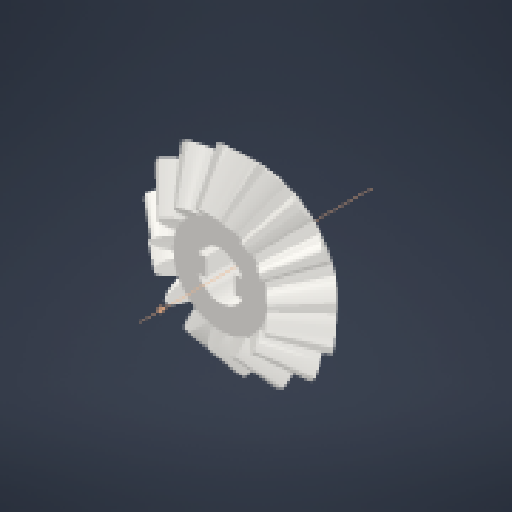
# Autodesk Inventor part: Bevel Gear2
Saved by Autodesk Inventor 2026 (Build 300175050, 175E)
## iProperties
CustomPartVersion: 1
Created: 2026-04-30
Part Number: Bevel Gear2
Material: Steel, Mild
Document SubType Name: Modeling
Designer: sniel
Categories: <?xml version="1.0" encoding="UTF-16"?> <MemberInstance><Categories><FamilyTemplate><FamilyTemplateParameter ValueType="xs:double" Id="1" ObjectReferenceKey="da_z" ObjectType="kUserParameterObject"/><FamilyTemplateParameter ValueType="xs:double" Id="2" ObjectReferenceKey="da_b" ObjectType="kUserParameterObject"/><FamilyTemplateParameter ValueType="xs:double" Id="3" ObjectReferenceKey="da_beta" ObjectType="kUserParameterObject"/><FamilyTemplateParameter ValueType="xs:double" Id="4" ObjectReferenceKey="da_dae" ObjectType="kUserParameterObject"/><FamilyTemplateParameter ValueType="xs:double" Id="5" ObjectReferenceKey="da_ve" ObjectType="kUserParameterObject"/><FamilyTemplateParameter ValueType="xs:double" Id="6" ObjectReferenceKey="da_omega" ObjectType="kUserParameterObject"/><FamilyTemplateParameter ValueType="xs:string" Id="7" ObjectReferenceKey="EAIAABAAAAAAHwAAAAAAAIAAAAAAAAAA" ObjectType="83914240" SubObjectId="SurfaceGeometry"/></FamilyTemplate><ParamToTemplateMap><ParamToTemplate CategoryParameter="//CategoryParameter[@InternalName='046C89C9-8512-4d59-83FE-43B91F4F132A']" TemplateParameter="1"/><ParamToTemplate CategoryParameter="//CategoryParameter[@InternalName='2552DF32-E462-4b46-AEBF-C6C7768E72AC']" TemplateParameter="2"/><ParamToTemplate CategoryParameter="//CategoryParameter[@InternalName='C9EE641D-15FC-4fae-A226-E94C4372FDD7']" TemplateParameter="3"/><ParamToTemplate><ParamToTemplate CategoryParameter="//CategoryParameter[@InternalName='00B6519A-459B-49c7-AD84-2E56D39A5744']" ConstantValue="-0.000000"/></ParamToTemplate><ParamToTemplate><ParamToTemplate CategoryParameter="//CategoryParameter[@InternalName='04B31F0E-C7A6-4894-AA32-9629BEFACF47']" ConstantValue="1.000000"/></ParamToTemplate><ParamToTemplate><ParamToTemplate CategoryParameter="//CategoryParameter[@InternalName='43CBEC2E-7847-49e7-A936-2F7889FCB2D9']" ConstantValue="0.200000"/></ParamToTemplate><ParamToTemplate><ParamToTemplate CategoryParameter="//CategoryParameter[@InternalName='B1EFC894-105D-4ebd-86BF-FA20ED196853']" ConstantValue="0.300000"/></ParamToTemplate><ParamToTemplate><ParamToTemplate CategoryParameter="//CategoryParameter[@InternalName='51175063-3D10-4879-93E8-6246FE8B403D']" ConstantValue="2060000000.000000"/></ParamToTemplate><ParamToTemplate><ParamToTemplate CategoryParameter="//CategoryParameter[@InternalName='A3A52E27-4454-46a9-B0BD-C932399B70AF']" ConstantValue="0.300000"/></ParamToTemplate><ParamToTemplate CategoryParameter="//CategoryParameter[@InternalName='2A200944-5A8C-41ca-B96E-8520D2E510F1']" TemplateParameter="4"/><ParamToTemplate><ParamToTemplate CategoryParameter="//CategoryParameter[@InternalName='1A637F62-92C8-44bc-B81F-10802510B579']" ConstantValue="1.982903"/></ParamToTemplate><ParamToTemplate CategoryParameter="//CategoryParameter[@InternalName='B52DD4BE-6863-48fb-BF58-89EF6F9EC65C']" TemplateParameter="5"/><ParamToTemplate><ParamToTemplate CategoryParameter="//CategoryParameter[@InternalName='3956BFF2-84D2-457d-93C2-9B0613DEBA67']" ConstantValue="0.820609"/></ParamToTemplate><ParamToTemplate CategoryParameter="//CategoryParameter[@InternalName='739CFA02-461B-4bf8-8049-181FCAD8B28F']" TemplateParameter="6"/><ParamToTemplate><ParamToTemplate CategoryParameter="//CategoryParameter[@InternalName='A27E999F-E2CE-4481-8A2A-EBF499C4C3C5']" ConstantValue="-0.000000"/></ParamToTemplate><ParamToTemplate><ParamToTemplate CategoryParameter="//CategoryParameter[@InternalName='9E1B4470-B2D3-4ff1-B813-535BB4CDF51A']" ConstantValue="3520000.000000"/></ParamToTemplate><ParamToTemplate><ParamToTemplate CategoryParameter="//CategoryParameter[@InternalName='F8452263-BFF6-458c-9FB1-07C4B99E95CD']" ConstantValue="11400000.000000"/></ParamToTemplate><ParamToTemplate><ParamToTemplate CategoryParameter="//CategoryParameter[@InternalName='3E3BB259-FD49-497f-8171-6EBC954A3479']" ConstantValue="2.000000"/></ParamToTemplate><ParamToTemplate CategoryParameter="//CategoryParameter[@InternalName='27C3BAF2-7550-4e4b-AE2C-0DB134B7D9B7']" TemplateParameter="7"/></ParamToTemplateMap><Category DisplayName="Gear" InternalName="DC85795E-93AB-48d5-8EEE-5A27447B64BD" Mnemonic="Gear"><CategoryParameter DisplayName="z" InternalName="046C89C9-8512-4d59-83FE-43B91F4F132A" Mnemonic="z"/><CategoryParameter DisplayName="b" InternalName="2552DF32-E462-4b46-AEBF-C6C7768E72AC" Mnemonic="b"/><CategoryParameter DisplayName="||b|" InternalName="C9EE641D-15FC-4fae-A226-E94C4372FDD7" Mnemonic="beta"/><CategoryParameter DisplayName="x" InternalName="00B6519A-459B-49c7-AD84-2E56D39A5744" Mnemonic="x"/><CategoryParameter DisplayName="a*" InternalName="04B31F0E-C7A6-4894-AA32-9629BEFACF47" Mnemonic="a"/><CategoryParameter DisplayName="c*" InternalName="43CBEC2E-7847-49e7-A936-2F7889FCB2D9" Mnemonic="c"/><CategoryParameter DisplayName="r|.f|*" InternalName="B1EFC894-105D-4ebd-86BF-FA20ED196853" Mnemonic="rf"/><CategoryParameter DisplayName="E" InternalName="51175063-3D10-4879-93E8-6246FE8B403D" Mnemonic="E"/><CategoryParameter DisplayName="||m|" InternalName="A3A52E27-4454-46a9-B0BD-C932399B70AF" Mnemonic="mi"/><Category DisplayName="BevelGear" InternalName="0C98F69A-0C2B-4791-B2FE-7691BB227E77" Mnemonic="BevelGear"><CategoryParameter DisplayName="d|.ae|" InternalName="2A200944-5A8C-41ca-B96E-8520D2E510F1" Mnemonic="dae"/><CategoryParameter DisplayName="d|.ai|" InternalName="1A637F62-92C8-44bc-B81F-10802510B579" Mnemonic="dai"/><CategoryParameter DisplayName="A|.e|" InternalName="B52DD4BE-6863-48fb-BF58-89EF6F9EC65C" Mnemonic="ve"/><CategoryParameter DisplayName="A|.i|" InternalName="3956BFF2-84D2-457d-93C2-9B0613DEBA67" Mnemonic="vi"/><CategoryParameter DisplayName="||S|" InternalName="739CFA02-461B-4bf8-8049-181FCAD8B28F" Mnemonic="omega"/><CategoryParameter DisplayName="x|.t|" InternalName="A27E999F-E2CE-4481-8A2A-EBF499C4C3C5" Mnemonic="xt"/><CategoryParameter DisplayName="||s||.Flim|" InternalName="9E1B4470-B2D3-4ff1-B813-535BB4CDF51A" Mnemonic="sFlim"/><CategoryParameter DisplayName="||s||.Hlim|" InternalName="F8452263-BFF6-458c-9FB1-07C4B99E95CD" Mnemonic="sHlim"/><CategoryParameter DisplayName="type" InternalName="3E3BB259-FD49-497f-8171-6EBC954A3479" Mnemonic="type"/><CategoryParameter DisplayName="PitchDiameter" InternalName="27C3BAF2-7550-4e4b-AE2C-0DB134B7D9B7" Mnemonic="IDS_PITCHDIAM"/></Category></Category></Categories></MemberInstance>
Mass: 60.9118 g
Surface Area: 34.3074 cm^2
Volume: 7.7496 cm^3
Density: 7.86 g/cm^3
Appearance: Steel
Author: sniel
Autodesk Inventor part; units mm, degrees
ref_plane "Mesh Plane2" through (0, 0, 0) normal (0.9781476, 0.2079117, 0) x (0, 0, 1)
sketch "Teeth Body Sketch" plane through (0, 0, 0) normal (1, 0, 0) x (0, 1, 0)
  line L0 (0, 0) -> (13.302944, -16.697056) construction
  line L1 (13.302944, -16.697056) -> (16.414214, -13.585786)
  line L2 (16.414214, -13.585786) -> (0, 0) construction
  line L3 (15, -15) -> (0, 0) construction
  line L4 (8.035247, -10.085359) -> (9.914517, -8.206089)
  line L5 (13.302944, -16.697056) -> (8.035247, -10.085359)
  line L6 (16.414214, -13.585786) -> (9.914517, -8.206089)
  line L7 (0, -39.386751) -> (0, 6.564458)
  line L8 (0, -15) -> (16.414214, -15) construction
  dimension "d0" = 30
  dimension "d1" = 26.60589
  dimension "d2" = 32.82843
  dimension "d3" = 8.4
  dimension "d4" = 13.58579
  constraints: 16 end point, 4 point on line, 3 perpendicular, 2 collinear, 1 horizontal alignment, 1 vertical alignment
  measures "d0" diameter of L3.start L7
  measures "d1" diameter of L0.end L7
  measures "d2" diameter of L1.end L7
  measures "d3" distance between parallel lines of L1 L4
  measures "d4" vertical distance of L1.end L0.start
revolve "Teeth Body" add sketch "Teeth Body Sketch" angle 360 about axis through (0, 0, 0) along (0, 0, 1)
ref_plane "Tooth Plane" through (0, 15, -15) normal (0, -0.7071068, 0.7071068) x (1, 0, 0)
sketch "Start Sketch" plane through (0, 15, -15) normal (0, -0.7071068, 0.7071068) x (1, 0, 0)
  line L0 (0, -23.505131) -> (0, 10.644758)
  arc A0 (-0.859413, -2.928) -> (-4.075674, 2.979088) centre (-8.774532, -3.408453) ccw
  arc A1 (4.075674, 2.979088) -> (0.859413, -2.928) centre (8.774532, -3.408453) ccw
  line L1 (-0.859413, -2.928) -> (0.859413, -2.928)
  arc A2 (4.075674, 2.979088) -> (-4.075674, 2.979088) centre (0, -21.213203) ccw
  dimension "d7" = 7.92969
  dimension "d8" = 8.77453
  dimension "d9" = 17.80475
  dimension "d57" = 24.5332
  dimension "d58" = 18.2852
  constraints: 6 point on circle, 3 centre point, 3 symmetric about line, 2 end point, 1 coincident, 1 perpendicular, 1 other
  measures "d7" radius of A0
  measures "d8" horizontal distance of point (0, -21.213) A0.centre
  measures "d9" vertical distance of point (0, -21.213) A0.centre
  measures "d57" radius of A2
  measures "d58" distance from line of A2.centre L1
sketch "End Sketch" plane through (0, 8.90474, -8.90474) normal (0, -0.7071068, 0.7071068) x (1, 0, 0)
  line L0 (0, -15.35404) -> (0, 6.953444)
  arc A0 (-0.51019, -1.738205) -> (-2.419521, 1.768533) centre (-5.208995, -2.023426) ccw
  arc A1 (2.419521, 1.768533) -> (0.51019, -1.738205) centre (5.208995, -2.023426) ccw
  line L1 (-0.51019, -1.738205) -> (0.51019, -1.738205)
  arc A2 (2.419521, 1.768533) -> (-2.419521, 1.768533) centre (0, -12.593203) ccw
  dimension "d12" = 4.70745
  dimension "d15" = 5.20899
  dimension "d16" = 10.56978
  dimension "d59" = 14.56412
  dimension "d60" = 10.855
  constraints: 6 point on circle, 3 centre point, 3 symmetric about line, 2 end point, 1 coincident, 1 other
  measures "d12" radius of A0
  measures "d15" horizontal distance of A0.centre point (0, -12.593)
  measures "d16" vertical distance of A0.centre point (0, -12.593)
  measures "d59" radius of A2
  measures "d60" distance from line of A2.centre L1
loft "Loft" cut profiles "Start Sketch", "End Sketch"
pattern_circular "Circular Pattern" count 15 over 360 about axis through (0, 0, 0) along (0, 0, 1) of "Loft"
ref_plane "End Plane" through (0, 8.90474, -8.90474) normal (0, -0.7071068, 0.7071068) x (1, 0, 0)
sketch3d "3D Sketch Right"
ref_plane "End Plane Right" through (-2.29609, 8.603625, -8.90474) normal (0.1823277, -0.6831959, 0.7071068) x (0.9661849, 0.2578504, 0)
sketch "End Sketch Right" plane through (-2.29609, 8.603625, -8.90474) normal (0.1823277, -0.6831959, 0.7071068) x (0.9661849, 0.2578504, 0)
  arc A0 (-0.51019, -1.738205) -> (-2.419521, 1.768533) centre (-5.208995, -2.023426) ccw
  line L0 (0, -19.114994) -> (0, 10.288445)
  arc A1 (2.419521, 1.768533) -> (0.51019, -1.738205) centre (5.208995, -2.023426) ccw
  line L1 (-0.51019, -1.738205) -> (0.51019, -1.738205)
  arc A2 (2.419521, 1.768533) -> (-2.419521, 1.768533) centre (0, -12.593203) ccw
  dimension "d70" = 5.20899
  dimension "d71" = 10.56978
  dimension "d72" = 4.70745
  dimension "d73" = 10.855
  dimension "d74" = 14.56412
  constraints: 6 point on circle, 3 centre point, 3 symmetric about line, 2 end point, 1 coincident, 1 perpendicular, 1 other
  measures "d70" horizontal distance of A2.centre A0.centre
  measures "d71" vertical distance of point (0, -12.593) A0.centre
  measures "d72" radius of A0
  measures "d73" distance from line of point (0, -12.593) L1
  measures "d74" radius of A2
feature "Loft Right" [suppressed]
pattern_circular "Circular Pattern Right" [suppressed]
sketch3d "3D Sketch Left"
ref_plane "End Plane Left" through (2.297938, 8.603625, -8.905436) normal (-0.1824624, -0.6831509, 0.7071155) x (0.9661332, -0.258044, 0)
sketch "End Sketch Left" plane through (2.297938, 8.603625, -8.905436) normal (-0.1824624, -0.6831509, 0.7071155) x (0.9661332, -0.258044, 0)
  line L0 (0, -32.194268) -> (0, 15.171544)
  arc A0 (-0.51019, -1.73805) -> (-2.419521, 1.768689) centre (-5.208995, -2.02327) ccw
  arc A1 (2.419521, 1.768689) -> (0.51019, -1.73805) centre (5.208995, -2.02327) ccw
  line L1 (-0.51019, -1.73805) -> (0.51019, -1.73805)
  ellipse E0 centre (0, -5.80251) end of major axis (9.914517, -5.80251) minor radius 7.010708
  arc A2 (2.419521, 1.768689) -> (-2.419521, 1.768689) centre (0, -12.593048) ccw
  dimension "d56" = 7.01071
  dimension "d30" = 4.70745
  dimension "d31" = 5.20899
  dimension "d32" = 10.56978
  dimension "d61" = 14.56412
  dimension "d62" = 10.855
  constraints: 6 point on circle, 3 centre point, 3 symmetric about line, 2 end point, 1 coincident, 2 other
  measures "d30" radius of A0
  measures "d31" horizontal distance of point (0, -12.593) A0.centre
  measures "d32" vertical distance of A0.centre point (0, -12.593)
  measures "d61" radius of A2
  measures "d62" distance from line of point (0, -12.593) L1
feature "Loft Left" [suppressed]
pattern_circular "Circular Pattern Left" [suppressed]
sketch "Body Sketch" plane through (0, 0, 0) normal (1, 0, 0) x (0, 1, 0)
  line L0 (0, -35.037536) -> (0, -19.530831)
  line L1 (13.302944, -16.697056) -> (8.035247, -10.085359)
  line L2 (8.035247, -10.085359) -> (0, -10.085359)
  line L3 (13.302944, -16.697056) -> (0, -16.697056)
  constraints: 4 end point, 2 perpendicular, 2 point on line
sketch "Body Sketch outline for Fix Body" plane through (0, 0, 0) normal (1, 0, 0) x (0, 1, 0)
  line L0 (0, -16.697056) -> (13.302944, -16.697056)
  line L1 (0, -10.085359) -> (0, -16.697056)
  line L2 (8.035247, -10.085359) -> (0, -10.085359)
  line L3 (13.302944, -16.697056) -> (8.035247, -10.085359)
revolve "Fix Body" add sketch "Body Sketch outline for Fix Body" angle 360 about axis through (0, 0, 0) along (0, 0, 1)
sketch "Sketch6" plane through (0, 0, 0) normal (1, 0, 0) x (0, 1, 0)
  line L0 (15, -15) -> (0, 0)
  line L1 (0, -37.799919) -> (0, 6.299986)
surface revolve "Pitch Diameter" sketch "Sketch6" angle 360 about axis through (0, 0, 0) along (0, 0, 1) shown no curves L0
sketch "Sketch8" plane through (0, 0, -16.697056) normal (0, 0, -1) x (-1, 0, 0)
  circle A0 centre (0, 0) radius 4
  line L0 (-5.5, -1.5) -> (-2.5, -1.5)
  line L1 (-2.5, -1.5) -> (-2.5, 1.5)
  line L2 (-2.5, 1.5) -> (-5.5, 1.5)
  line L3 (-5.5, 1.5) -> (-5.5, -1.5)
  line L4 (-5.5, -1.5) -> (-2.5, 1.5) construction
  line L5 (-2.5, -1.5) -> (-5.5, 1.5) construction
  line L6 (2.5, -1.5) -> (5.5, -1.5)
  line L7 (5.5, -1.5) -> (5.5, 1.5)
  line L8 (5.5, 1.5) -> (2.5, 1.5)
  line L9 (2.5, 1.5) -> (2.5, -1.5)
  line L10 (2.5, -1.5) -> (5.5, 1.5) construction
  line L11 (5.5, -1.5) -> (2.5, 1.5) construction
  point P0 (-4, 0)
  point P1 (4, 0)
  point P2 (-3.708099, -1.5)
  point P3 (3.708099, -1.5)
  point P4 (3.708099, 1.5)
  point P5 (-3.708099, 1.5)
  dimension "d94" = 8
  dimension "d95" = 3
  dimension "d96" = 3
  dimension "d97" = 3
  dimension "d98" = 3
  constraints: 24 end point, 4 midpoint, 4 parallel, 2 horizontal, 2 perpendicular, 2 point on circle, 1 centre point, 1 coincident
  measures "d94" diameter of A0
  measures "d95" distance of L2.end L1.end
  measures "d96" distance of L1.end L0.end
  measures "d97" distance of L8.end L7.end
  measures "d98" distance of L7.end L6.end
extrude "Extrusion1" cut sketch "Sketch8" against normal blind 11.5 contours L8 L9 L6 A0 L0 L1 L2
equation "\"d0\" = da_de"
equation "\"d1\" = da_dfe"
equation "\"d2\" = da_dae"
equation "\"d3\" = da_b"
equation "\"d4\" = da_ve"
equation "\"d7\" = fd_rr"
equation "\"d8\" = fd_x"
equation "\"d9\" = fd_y"
equation "\"d57\" = 0.5 * fd_dva + 0.3 * da_he"
equation "\"d58\" = 0.5 * fd_dva - 1.12 * da_he"
equation "\"da_teethtype\" = 0"
equation "\"da_b\" = 8.4"
equation "\"da_de\" = 30"
equation "\"da_dae\" = 32.82843"
equation "\"da_dfe\" = 26.60589"
equation "\"da_le\" = 21.2132"
equation "\"da_omega\" = 90deg"
equation "\"da_beta\" = 0"
equation "\"da_delta\" = 45deg"
equation "\"da_alpha\" = 20deg"
equation "\"da_he\" = 4.4"
equation "\"da_ve\" = 13.58579"
equation "\"da_zv\" = 21.213203"
equation "\"fd_loft\" = da_b + 0.05 * da_he"
equation "\"fd_x\" = fd_x1 + fd_x2"
equation "\"fd_y\" = fd_y1 - fd_y2"
equation "\"fd_dd\" = fd_dva - 0.8 * da_he"
equation "\"da_dvw\" = 42.42641"
equation "\"d11\" = fd_loft"
equation "\"da_dm\" = 24.0603"
equation "\"da_x\" = 0"
equation "\"da_m\" = 2"
equation "\"d50\" = da_omega"
equation "\"fd_rr\" = 7.929687"
equation "\"fd_dva\" = 46.426407"
equation "\"fd_x1\" = 1.586766"
equation "\"fd_x2\" = 7.187766"
equation "\"fd_y1\" = 21.153774"
equation "\"fd_y2\" = 3.349024"
body "Solid1"
body "Srf1"
